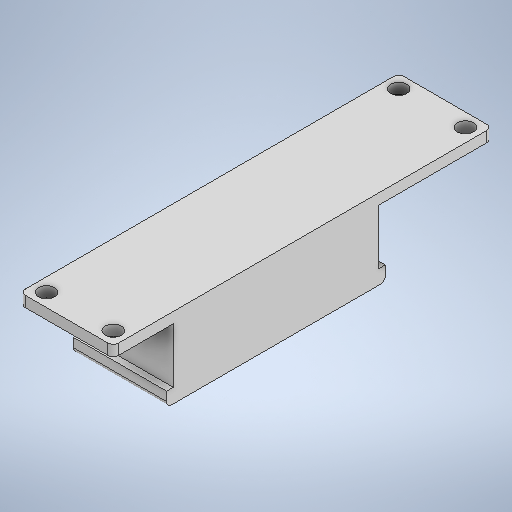
# Autodesk Inventor part: Relais_Platte
Saved by Autodesk Inventor 2025.2 (Build 292293000, 293)
## iProperties
Created: 2025-03-23
Part Number: Relais_Platte
Material: Generisch
Document SubType Name: Modeling
Designer: Quatana
Density: 1 g/cm^3
Appearance: Vorgabe
Author: Quatana
## iProperties of the stored document Relais_Platte_3D-Druck.ipt
Created: 2025-03-23
Part Number: Relais_Platte_3D-Druck
Material: Generisch
Document SubType Name: Modeling
Designer: Quatana
Density: 1 g/cm^3
Appearance: Vorgabe
Author: Quatana
Autodesk Inventor part; units mm, degrees
ref_plane "YZ Plane" through (0, 0, 0) normal (1, 0, 0) x (0, 1, 0)
ref_plane "XZ Plane" through (0, 0, 0) normal (0, 1, 0) x (-1, 0, 0)
ref_plane "XY Plane" through (0, 0, 0) normal (0, 0, 1) x (1, 0, 0)
sketch "Skizze1" plane through (0, 0, 0) normal (0, 0, 1) x (1, 0, 0)
  line L0 (-8.75, -35.5) -> (8.75, -35.5)
  line L1 (8.75, -35.5) -> (8.75, 35.5)
  line L2 (8.75, 35.5) -> (-8.75, 35.5)
  line L3 (-8.75, 35.5) -> (-8.75, -35.5)
  line L4 (-8.75, -35.5) -> (8.75, 35.5) construction
  line L5 (8.75, -35.5) -> (-8.75, 35.5) construction
  point P0 (0, 0)
  dimension "d0" = 17.5
  dimension "d1" = 71
  constraints: 12 end point, 2 midpoint, 2 parallel, 1 horizontal, 1 perpendicular
  measures "d0" distance of L2.end L1.end
  measures "d1" distance of L1.end L0.end
extrude "Extrusion1" add sketch "Skizze1" along normal blind 2
sketch "Skizze2" plane through (0, 0, 2) normal (0, 0, 1) x (1, 0, 0)
  circle A0 centre (-6.25, 33) radius 1.5
  line L0 (8.75, 35.5) -> (-8.75, 35.5) projected
  line L1 (0, 35.5) -> (0, 32.4568) construction
  circle A1 centre (6.25, 33) radius 1.5
  line L2 (-3.3034, 0) -> (2.2681, 0) construction
  circle A2 centre (-6.25, -33) radius 1.5
  circle A3 centre (6.25, -33) radius 1.5
  line L3 (-8.75, 35.5) -> (-8.75, -35.5) construction
  point P0 (0, 0)
  dimension "d4" = 3
  dimension "d5" = 2.5
  dimension "d6" = 2.5
  constraints: 4 centre point, 4 end point, 3 symmetric about line, 1 horizontal, 1 midpoint, 1 vertical, 3 other
  measures "d4" diameter of A0
  measures "d5" distance from line of L0 A0.centre
  measures "d6" distance from line of L3 A0.centre
extrude "Extrusion2" cut sketch "Skizze2" against normal blind 2
sketch "Skizze3" plane through (0, 0, 0) normal (0, 0, -1) x (-1, 0, 0)
  line L0 (8.75, 35.5) -> (8.75, -35.5) projected
  line L1 (-8.75, -25.5) -> (8.75, -25.5)
  line L2 (8.75, -25.5) -> (8.75, 15.5)
  line L3 (8.75, 15.5) -> (-8.75, 15.5)
  line L4 (-8.75, 15.5) -> (-8.75, -25.5)
  line L5 (-8.75, -25.5) -> (8.75, 15.5) construction
  line L6 (8.75, -25.5) -> (-8.75, 15.5) construction
  line L7 (8.75, -35.5) -> (-8.75, -35.5) projected
  line L8 (-8.75, -35.5) -> (-8.75, 35.5) projected
  point P0 (0, -5)
  point P1 (8.75, -25.5)
  dimension "d9" = 41
  dimension "d17" = 10
  constraints: 12 end point, 2 midpoint, 2 parallel, 1 horizontal, 1 perpendicular, 1 point on line, 1 vertical alignment
  measures "d9" distance between parallel lines of L1 L3
  measures "d17" distance between parallel lines of L7 L1
extrude "Extrusion3" add sketch "Skizze3" along normal blind 13 contours L0 L1 L4 L3
sketch "Skizze4" plane through (-8.75, -35.5, 2) normal (-1, 0, 0) x (0, 0, 1)
  line L0 (-2, 10) -> (-15, 10) projected
  line L1 (-12.32, 10) -> (-2, 10)
  line L2 (-2, 10) -> (-2, 11.25)
  line L3 (-2, 11.25) -> (-12.32, 11.25)
  line L4 (-12.32, 11.25) -> (-12.32, 10)
  line L5 (-15, 10) -> (-15, 51) projected
  line L6 (-4.404, 30.5) -> (2.981, 30.5) construction
  line L7 (-2, 51) -> (-15, 51)
  line L8 (-2, 51) -> (-2, 49.75)
  line L9 (-2, 49.75) -> (-12.32, 49.75)
  line L10 (-12.32, 49.75) -> (-12.32, 51)
  line L11 (-2, 10) -> (-12.32, 10)
  point P0 (-2, 35.5)
  point P1 (-12.32, 10.625)
  dimension "d12" = 2.68
  dimension "d13" = 1.25
  constraints: 20 end point, 5 symmetric about line, 3 point on line, 2 horizontal, 2 parallel, 1 collinear, 1 midpoint, 1 perpendicular
  measures "d12" distance from line of L5 point (-12.32, 10.625)
  measures "d13" distance between parallel lines of L3 L0
extrude "Extrusion4" cut sketch "Skizze4" against normal blind 17.5
fillet "Rundung1" radius 1 6 edges at (-8.75, -35.5, 1) (8.75, -35.5, 1) (8.75, 35.5, 1) (-8.75, 35.5, 1) (0, 15.5, -13) (0, -25.5, -13)
